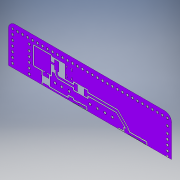
# Autodesk Inventor part: BaseBandAmp_Top_SolderMaskUpper
Saved by Autodesk Inventor 2018 (Build 220112000, 112)
## iProperties
Created: 2018-03-29
Part Number: BaseBandAmp_Top_SolderMaskUpper
Material: Generic
Document SubType Name: Modeling
Designer: Eric Weeks
Density: 1 g/cm^3
Appearance: Default
Author: Eric Weeks
Autodesk Inventor part; units mm, degrees
(part 1 of 2)
ref_plane "YZ Plane" through (0, 0, 0) normal (1, 0, 0) x (0, 1, 0)
ref_plane "XZ Plane" through (0, 0, 0) normal (0, 1, 0) x (-1, 0, 0)
ref_plane "XY Plane" through (0, 0, 0) normal (0, 0, 1) x (1, 0, 0)
sketch "Sketch1" plane through (0, 0, 0) normal (0, 0, 1) x (1, 0, 0)
  line L0 (3476.498, -1500.378) -> (3473.6532, -1500.378) projected
  line L1 (3473.6532, -1500.378) -> (3473.6532, -1503.3396) projected
  line L2 (3473.6532, -1503.3396) -> (3473.9326, -1503.6038) projected
  line L3 (3473.9326, -1503.6038) -> (3477.133, -1503.6038) projected
  line L4 (3477.133, -1503.6038) -> (3478.3268, -1503.1136) projected
  line L5 (3478.3268, -1503.1136) -> (3479.2412, -1502.2043) projected
  line L6 (3479.2412, -1502.2043) -> (3479.7238, -1501.0206) projected
  line L7 (3479.7238, -1501.0206) -> (3479.7238, -1494.0001) projected
  line L8 (3479.7238, -1494.0001) -> (3479.4698, -1493.7359) projected
  line L9 (3479.4698, -1493.7359) -> (3476.498, -1493.7359) projected
  line L10 (3476.498, -1493.7359) -> (3476.498, -1500.378) projected
  line L11 (3455.4922, -1494.0001) -> (3455.4922, -1501.0206) projected
  line L12 (3455.4922, -1501.0206) -> (3455.9748, -1502.2043) projected
  line L13 (3455.9748, -1502.2043) -> (3456.8892, -1503.1136) projected
  line L14 (3456.8892, -1503.1136) -> (3458.083, -1503.6038) projected
  line L15 (3458.083, -1503.6038) -> (3461.2834, -1503.6038) projected
  line L16 (3461.2834, -1503.6038) -> (3461.5374, -1503.3396) projected
  line L17 (3461.5374, -1503.3396) -> (3461.5374, -1500.378) projected
  line L18 (3461.5374, -1500.378) -> (3458.718, -1500.378) projected
  line L19 (3458.718, -1500.378) -> (3458.718, -1493.7359) projected
  line L20 (3458.718, -1493.7359) -> (3455.7462, -1493.7359) projected
  line L21 (3455.7462, -1493.7359) -> (3455.4922, -1494.0001) projected
  line L22 (3770.6966, -1575.7959) -> (3770.9348, -1574.6146) projected
  line L23 (3770.9348, -1574.6146) -> (3770.9348, -1567.3146) projected
  line L24 (3770.9348, -1567.3146) -> (3770.503, -1565.1734) projected
  line L25 (3770.503, -1565.1734) -> (3769.3854, -1563.4919) projected
  line L26 (3769.3854, -1563.4919) -> (3767.709, -1562.3692) projected
  line L27 (3767.709, -1562.3692) -> (3765.5754, -1561.9425) projected
  line L28 (3765.5754, -1561.9425) -> (3756.9902, -1561.9425) projected
  line L29 (3756.9902, -1561.9425) -> (3754.8566, -1562.3692) projected
  line L30 (3754.8566, -1562.3692) -> (3754.755, -1562.4378) projected
  line L31 (3754.755, -1562.4378) -> (3754.5772, -1562.5166) projected
  line L32 (3754.5772, -1562.5166) -> (3754.3994, -1562.6131) projected
  line L33 (3754.3994, -1562.6131) -> (3754.3232, -1562.6283) projected
  line L34 (3754.3232, -1562.6283) -> (3754.247, -1562.6639) projected
  line L35 (3754.247, -1562.6639) -> (3754.0438, -1562.6766) projected
  line L36 (3754.0438, -1562.6766) -> (3753.866, -1562.7096) projected
  line L37 (3753.866, -1562.7096) -> (3749.3448, -1562.7096) projected
  line L38 (3749.3448, -1562.7096) -> (3749.167, -1562.6766) projected
  line L39 (3749.167, -1562.6766) -> (3748.9638, -1562.6639) projected
  line L40 (3748.9638, -1562.6639) -> (3748.8876, -1562.6283) projected
  line L41 (3748.8876, -1562.6283) -> (3748.8114, -1562.6131) projected
  line L42 (3748.8114, -1562.6131) -> (3748.6336, -1562.5166) projected
  line L43 (3748.6336, -1562.5166) -> (3748.4558, -1562.4378) projected
  line L44 (3748.4558, -1562.4378) -> (3748.3542, -1562.3692) projected
  line L45 (3748.3542, -1562.3692) -> (3746.2206, -1561.9425) projected
  line L46 (3746.2206, -1561.9425) -> (3737.6354, -1561.9425) projected
  line L47 (3737.6354, -1561.9425) -> (3735.5018, -1562.3692) projected
  line L48 (3735.5018, -1562.3692) -> (3735.4002, -1562.4378) projected
  line L49 (3735.4002, -1562.4378) -> (3735.2224, -1562.5166) projected
  line L50 (3735.2224, -1562.5166) -> (3735.0446, -1562.6131) projected
  line L51 (3735.0446, -1562.6131) -> (3734.9684, -1562.6283) projected
  line L52 (3734.9684, -1562.6283) -> (3734.8922, -1562.6639) projected
  line L53 (3734.8922, -1562.6639) -> (3734.689, -1562.6766) projected
  line L54 (3734.689, -1562.6766) -> (3734.5112, -1562.7096) projected
  line L55 (3734.5112, -1562.7096) -> (3704.844, -1562.7096) projected
  line L56 (3704.844, -1562.7096) -> (3704.59, -1562.6639) projected
  line L57 (3704.59, -1562.6639) -> (3704.336, -1562.6232) projected
  line L58 (3704.336, -1562.6232) -> (3704.3106, -1562.6156) projected
  line L59 (3704.3106, -1562.6156) -> (3704.2852, -1562.6131) projected
  line L60 (3704.2852, -1562.6131) -> (3704.0566, -1562.481) projected
  line L61 (3704.0566, -1562.481) -> (3703.828, -1562.354) projected
  line L62 (3703.828, -1562.354) -> (3703.828, -1562.3413) projected
  line L63 (3703.828, -1562.3413) -> (3703.8026, -1562.3311) projected
  line L64 (3703.8026, -1562.3311) -> (3703.6502, -1562.1305) projected
  line L65 (3703.6502, -1562.1305) -> (3703.4724, -1561.9324) projected
  line L66 (3703.4724, -1561.9324) -> (3703.447, -1561.9171) projected
  line L67 (3703.447, -1561.9171) -> (3703.447, -1561.9019) projected
  line L68 (3703.447, -1561.9019) -> (3703.3708, -1561.6555) projected
  line L69 (3703.3708, -1561.6555) -> (3703.2692, -1561.4117) projected
  line L70 (3703.2692, -1561.4117) -> (3703.1676, -1560.9189) projected
  line L71 (3703.1676, -1560.9189) -> (3702.05, -1559.2374) projected
  line L72 (3702.05, -1559.2374) -> (3700.3736, -1558.1147) projected
  line L73 (3700.3736, -1558.1147) -> (3700.0434, -1558.0512) projected
  line L74 (3700.0434, -1558.0512) -> (3699.9418, -1558.0131) projected
  line L75 (3699.9418, -1558.0131) -> (3699.8402, -1557.9979) projected
  line L76 (3699.8402, -1557.9979) -> (3699.6878, -1557.9115) projected
  line L77 (3699.6878, -1557.9115) -> (3699.5354, -1557.848) projected
  line L78 (3699.5354, -1557.848) -> (3699.4338, -1557.7795) projected
  line L79 (3699.4338, -1557.7795) -> (3699.3576, -1557.7287) projected
  line L80 (3699.3576, -1557.7287) -> (3699.2306, -1557.5966) projected
  line L81 (3699.2306, -1557.5966) -> (3699.1036, -1557.4797) projected
  line L82 (3699.1036, -1557.4797) -> (3699.0528, -1557.3858) projected
  line L83 (3699.0528, -1557.3858) -> (3698.9766, -1557.307) projected
  line L84 (3698.9766, -1557.307) -> (3698.9258, -1557.1419) projected
  line L85 (3698.9258, -1557.1419) -> (3698.8242, -1556.9895) projected
  line L86 (3698.8242, -1556.9895) -> (3698.8242, -1556.8828) projected
  line L87 (3698.8242, -1556.8828) -> (3698.7734, -1556.7838) projected
  line L88 (3698.7734, -1556.7838) -> (3698.0876, -1553.3294) projected
  line L89 (3698.0876, -1553.3294) -> (3696.6398, -1551.1551) projected
  line L90 (3696.6398, -1551.1551) -> (3696.2588, -1550.5989) projected
  line L91 (3696.2588, -1550.5989) -> (3695.7, -1550.2255) projected
  line L92 (3695.7, -1550.2255) -> (3695.5984, -1550.1163) projected
  line L93 (3695.5984, -1550.1163) -> (3695.4714, -1550.0248) projected
  line L94 (3695.4714, -1550.0248) -> (3659.632, -1514.2007) projected
  line L95 (3659.632, -1514.2007) -> (3659.5558, -1514.0711) projected
  line L96 (3659.5558, -1514.0711) -> (3659.4288, -1513.9568) projected
  line L97 (3659.4288, -1513.9568) -> (3659.0732, -1513.4006) projected
  line L98 (3659.0732, -1513.4006) -> (3656.33, -1511.5769) projected
  line L99 (3656.33, -1511.5769) -> (3653.7646, -1511.0663) projected
  line L100 (3653.7646, -1511.0663) -> (3653.1042, -1510.9342) projected
  line L101 (3653.1042, -1510.9342) -> (3652.4692, -1511.0663) projected
  line L102 (3652.4692, -1511.0663) -> (3652.2914, -1511.0689) projected
  line L103 (3652.2914, -1511.0689) -> (3652.139, -1511.0968) projected
  line L104 (3652.139, -1511.0968) -> (3544.824, -1511.0968) projected
  line L105 (3544.824, -1511.0968) -> (3544.6716, -1511.0714) projected
  line L106 (3544.6716, -1511.0714) -> (3544.5446, -1511.0714) projected
  line L107 (3544.5446, -1511.0714) -> (3544.3922, -1511.0231) projected
  line L108 (3544.3922, -1511.0231) -> (3544.2652, -1511.0003) projected
  line L109 (3544.2652, -1511.0003) -> (3544.1382, -1510.9292) projected
  line L110 (3544.1382, -1510.9292) -> (3544.0112, -1510.8809) projected
  line L111 (3544.0112, -1510.8809) -> (3543.9096, -1510.7895) projected
  line L112 (3543.9096, -1510.7895) -> (3543.7826, -1510.7183) projected
  line L113 (3543.7826, -1510.7183) -> (3543.681, -1510.6117) projected
  line L114 (3543.681, -1510.6117) -> (3543.5794, -1510.5202) projected
  line L115 (3543.5794, -1510.5202) -> (3543.5032, -1510.3983) projected
  line L116 (3543.5032, -1510.3983) -> (3543.427, -1510.2891) projected
  line L117 (3543.427, -1510.2891) -> (3543.3762, -1510.157) projected
  line L118 (3543.3762, -1510.157) -> (3543.3, -1510.0351) projected
  line L119 (3543.3, -1510.0351) -> (3543.2746, -1509.8954) projected
  line L120 (3543.2746, -1509.8954) -> (3543.2238, -1509.7633) projected
  line L121 (3543.2238, -1509.7633) -> (3543.2238, -1509.6236) projected
  line L122 (3543.2238, -1509.6236) -> (3543.1984, -1509.4839) projected
  line L123 (3543.1984, -1509.4839) -> (3543.1984, -1508.0818) projected
  line L124 (3543.1984, -1508.0818) -> (3542.7666, -1505.9406) projected
  line L125 (3542.7666, -1505.9406) -> (3541.649, -1504.2591) projected
  line L126 (3541.649, -1504.2591) -> (3539.9726, -1503.1364) projected
  line L127 (3539.9726, -1503.1364) -> (3537.839, -1502.7097) projected
  line L128 (3537.839, -1502.7097) -> (3525.4438, -1502.7097) projected
  line L129 (3525.4438, -1502.7097) -> (3523.0308, -1503.1923) projected
  line L130 (3523.0308, -1503.1923) -> (3522.8784, -1503.1949) projected
  line L131 (3522.8784, -1503.1949) -> (3522.726, -1503.2228) projected
  line L132 (3522.726, -1503.2228) -> (3502.4568, -1503.2228) projected
  line L133 (3502.4568, -1503.2228) -> (3502.3044, -1503.1949) projected
  line L134 (3502.3044, -1503.1949) -> (3502.152, -1503.1923) projected
  line L135 (3502.152, -1503.1923) -> (3499.739, -1502.7097) projected
  line L136 (3499.739, -1502.7097) -> (3487.3438, -1502.7097) projected
  line L137 (3487.3438, -1502.7097) -> (3485.2102, -1503.1364) projected
  line L138 (3485.2102, -1503.1364) -> (3483.5338, -1504.2591) projected
  line L139 (3483.5338, -1504.2591) -> (3482.4162, -1505.9406) projected
  line L140 (3482.4162, -1505.9406) -> (3481.9844, -1508.0818) projected
  line L141 (3481.9844, -1508.0818) -> (3481.9844, -1509.4839) projected
  line L142 (3481.9844, -1509.4839) -> (3481.959, -1509.6236) projected
  line L143 (3481.959, -1509.6236) -> (3481.959, -1509.7633) projected
  line L144 (3481.959, -1509.7633) -> (3481.9082, -1509.8954) projected
  line L145 (3481.9082, -1509.8954) -> (3481.8828, -1510.0351) projected
  line L146 (3481.8828, -1510.0351) -> (3481.8066, -1510.157) projected
  line L147 (3481.8066, -1510.157) -> (3481.7558, -1510.2891) projected
  line L148 (3481.7558, -1510.2891) -> (3481.6796, -1510.3983) projected
  line L149 (3481.6796, -1510.3983) -> (3481.6034, -1510.5202) projected
  line L150 (3481.6034, -1510.5202) -> (3481.5018, -1510.6117) projected
  line L151 (3481.5018, -1510.6117) -> (3481.4002, -1510.7183) projected
  line L152 (3481.4002, -1510.7183) -> (3481.2732, -1510.7895) projected
  line L153 (3481.2732, -1510.7895) -> (3481.1716, -1510.8809) projected
  line L154 (3481.1716, -1510.8809) -> (3481.0446, -1510.9292) projected
  line L155 (3481.0446, -1510.9292) -> (3480.9176, -1511.0003) projected
  line L156 (3480.9176, -1511.0003) -> (3480.7906, -1511.0231) projected
  line L157 (3480.7906, -1511.0231) -> (3480.6382, -1511.0714) projected
  line L158 (3480.6382, -1511.0714) -> (3480.5112, -1511.0714) projected
  line L159 (3480.5112, -1511.0714) -> (3480.3588, -1511.0968) projected
  line L160 (3480.3588, -1511.0968) -> (3453.2062, -1511.0968) projected
  line L161 (3453.2062, -1511.0968) -> (3453.0792, -1511.0714) projected
  line L162 (3453.0792, -1511.0714) -> (3452.9268, -1511.0714) projected
  line L163 (3452.9268, -1511.0714) -> (3452.7998, -1511.0231) projected
  line L164 (3452.7998, -1511.0231) -> (3452.6728, -1511.0003) projected
  line L165 (3452.6728, -1511.0003) -> (3452.5458, -1510.9292) projected
  line L166 (3452.5458, -1510.9292) -> (3452.4188, -1510.8809) projected
  line L167 (3452.4188, -1510.8809) -> (3452.2918, -1510.7895) projected
  line L168 (3452.2918, -1510.7895) -> (3452.1902, -1510.7183) projected
  line L169 (3452.1902, -1510.7183) -> (3452.0886, -1510.6117) projected
  line L170 (3452.0886, -1510.6117) -> (3451.987, -1510.5202) projected
  line L171 (3451.987, -1510.5202) -> (3451.9108, -1510.3983) projected
  line L172 (3451.9108, -1510.3983) -> (3451.8346, -1510.2891) projected
  line L173 (3451.8346, -1510.2891) -> (3451.7838, -1510.157) projected
  line L174 (3451.7838, -1510.157) -> (3451.7076, -1510.0351) projected
  line L175 (3451.7076, -1510.0351) -> (3451.6822, -1509.8954) projected
  line L176 (3451.6822, -1509.8954) -> (3451.6314, -1509.7633) projected
  line L177 (3451.6314, -1509.7633) -> (3451.6314, -1509.6236) projected
  line L178 (3451.6314, -1509.6236) -> (3451.606, -1509.4839) projected
  line L179 (3451.606, -1509.4839) -> (3451.606, -1461.4474) projected
  line L180 (3451.606, -1461.4474) -> (3451.5806, -1461.3128) projected
  line L181 (3451.5806, -1461.3128) -> (3451.4536, -1461.2874) projected
  line L182 (3451.4536, -1461.2874) -> (3403.2698, -1461.2874) projected
  line L183 (3403.2698, -1461.2874) -> (3403.0158, -1461.2417) projected
  line L184 (3403.0158, -1461.2417) -> (3402.7618, -1461.201) projected
  line L185 (3402.7618, -1461.201) -> (3402.7364, -1461.1934) projected
  line L186 (3402.7364, -1461.1934) -> (3402.711, -1461.1909) projected
  line L187 (3402.711, -1461.1909) -> (3402.4824, -1461.0588) projected
  line L188 (3402.4824, -1461.0588) -> (3402.2538, -1460.9318) projected
  line L189 (3402.2538, -1460.9318) -> (3402.2538, -1460.9191) projected
  line L190 (3402.2538, -1460.9191) -> (3402.2284, -1460.9089) projected
  line L191 (3402.2284, -1460.9089) -> (3402.076, -1460.7083) projected
  line L192 (3402.076, -1460.7083) -> (3401.8982, -1460.5102) projected
  line L193 (3401.8982, -1460.5102) -> (3401.8728, -1460.4949) projected
  line L194 (3401.8728, -1460.4949) -> (3401.8728, -1460.4797) projected
  line L195 (3401.8728, -1460.4797) -> (3401.7712, -1460.2333) projected
  line L196 (3401.7712, -1460.2333) -> (3401.695, -1459.9895) projected
  line L197 (3401.695, -1459.9895) -> (3401.5426, -1459.3062) projected
  line L198 (3401.5426, -1459.3062) -> (3400.425, -1457.6247) projected
  line L199 (3400.425, -1457.6247) -> (3398.7486, -1456.502) projected
  line L200 (3398.7486, -1456.502) -> (3396.615, -1456.0753) projected
  line L201 (3396.615, -1456.0753) -> (3332.4038, -1456.0753) projected
  line L202 (3332.4038, -1456.0753) -> (3330.2702, -1456.502) projected
  line L203 (3330.2702, -1456.502) -> (3328.5938, -1457.6247) projected
  line L204 (3328.5938, -1457.6247) -> (3327.4762, -1459.3062) projected
  line L205 (3327.4762, -1459.3062) -> (3327.0444, -1461.4474) projected
  line L206 (3327.0444, -1461.4474) -> (3327.0444, -1525.6434) projected
  line L207 (3327.0444, -1525.6434) -> (3327.4762, -1527.7846) projected
  line L208 (3327.4762, -1527.7846) -> (3328.5938, -1529.4661) projected
  line L209 (3328.5938, -1529.4661) -> (3330.2702, -1530.5888) projected
  line L210 (3330.2702, -1530.5888) -> (3332.4038, -1531.0155) projected
  line L211 (3332.4038, -1531.0155) -> (3359.15, -1531.0155) projected
  line L212 (3359.15, -1531.0155) -> (3359.3024, -1531.0383) projected
  line L213 (3359.3024, -1531.0383) -> (3359.4294, -1531.0383) projected
  line L214 (3359.4294, -1531.0383) -> (3359.5818, -1531.0866) projected
  line L215 (3359.5818, -1531.0866) -> (3359.7088, -1531.112) projected
  line L216 (3359.7088, -1531.112) -> (3359.8358, -1531.1831) projected
  line L217 (3359.8358, -1531.1831) -> (3359.9628, -1531.2314) projected
  line L218 (3359.9628, -1531.2314) -> (3360.0644, -1531.3203) projected
  line L219 (3360.0644, -1531.3203) -> (3360.1914, -1531.3914) projected
  line L220 (3360.1914, -1531.3914) -> (3360.293, -1531.5006) projected
  line L221 (3360.293, -1531.5006) -> (3360.3946, -1531.5895) projected
  line L222 (3360.3946, -1531.5895) -> (3360.4708, -1531.714) projected
  line L223 (3360.4708, -1531.714) -> (3360.547, -1531.8207) projected
  line L224 (3360.547, -1531.8207) -> (3360.5978, -1531.9527) projected
  line L225 (3360.5978, -1531.9527) -> (3360.674, -1532.0747) projected
  line L226 (3360.674, -1532.0747) -> (3360.6994, -1532.2144) projected
  line L227 (3360.6994, -1532.2144) -> (3360.7502, -1532.3464) projected
  line L228 (3360.7502, -1532.3464) -> (3360.7502, -1532.4887) projected
  line L229 (3360.7502, -1532.4887) -> (3360.7756, -1532.6284) projected
  line L230 (3360.7756, -1532.6284) -> (3360.7756, -1541.9756) projected
  line L231 (3360.7756, -1541.9756) -> (3361.2582, -1544.3962) projected
  line L232 (3361.2582, -1544.3962) -> (3361.2582, -1544.5537) projected
  line L233 (3361.2582, -1544.5537) -> (3361.2836, -1544.7112) projected
  line L234 (3361.2836, -1544.7112) -> (3361.2836, -1564.96) projected
  line L235 (3361.2836, -1564.96) -> (3361.2582, -1565.1175) projected
  line L236 (3361.2582, -1565.1175) -> (3361.2582, -1565.275) projected
  line L237 (3361.2582, -1565.275) -> (3360.7756, -1567.6956) projected
  line L238 (3360.7756, -1567.6956) -> (3360.7756, -1575.7959) projected
  line L239 (3410.458, -1480.693) -> (3410.458, -1467.358) projected
  line L240 (3410.458, -1467.358) -> (3428.238, -1467.358) projected
  line L241 (3428.238, -1467.358) -> (3428.238, -1500.378) projected
  line L242 (3428.238, -1500.378) -> (3422.523, -1500.378) projected
  line L243 (3422.523, -1500.378) -> (3422.523, -1511.5845) projected
  line L244 (3422.523, -1511.5845) -> (3427.1204, -1516.1768) projected
  line L245 (3427.1204, -1516.1768) -> (3487.1914, -1516.1768) projected
  line L246 (3487.1914, -1516.1768) -> (3487.1914, -1507.9218) projected
  line L247 (3487.1914, -1507.9218) -> (3499.8914, -1507.9218) projected
  line L248 (3499.8914, -1507.9218) -> (3499.8914, -1530.7818) projected
  line L249 (3499.8914, -1530.7818) -> (3487.1914, -1530.7818) projected
  line L250 (3487.1914, -1530.7818) -> (3487.1914, -1522.5268) projected
  line L251 (3487.1914, -1522.5268) -> (3425.7234, -1522.5268) projected
  line L252 (3425.7234, -1522.5268) -> (3425.6726, -1522.5141) projected
  line L253 (3425.6726, -1522.5141) -> (3425.5202, -1522.5268) projected
  line L254 (3425.5202, -1522.5268) -> (3425.1138, -1522.4201) projected
  line L255 (3425.1138, -1522.4201) -> (3424.7074, -1522.3465) projected
  line L256 (3424.7074, -1522.3465) -> (3424.5804, -1522.2753) projected
  line L257 (3424.5804, -1522.2753) -> (3424.4534, -1522.2398) projected
  line L258 (3424.4534, -1522.2398) -> (3424.1232, -1522.001) projected
  line L259 (3424.1232, -1522.001) -> (3423.7422, -1521.7927) projected
  line L260 (3423.7422, -1521.7927) -> (3423.666, -1521.6861) projected
  line L261 (3423.666, -1521.6861) -> (3423.6152, -1521.6454) projected
  line L262 (3423.6152, -1521.6454) -> (3417.062, -1515.0973) projected
  line L263 (3417.062, -1515.0973) -> (3417.0112, -1515.0389) projected
  line L264 (3417.0112, -1515.0389) -> (3416.9096, -1514.95) projected
  line L265 (3416.9096, -1514.95) -> (3416.7064, -1514.5893) projected
  line L266 (3416.7064, -1514.5893) -> (3416.4524, -1514.2464) projected
  line L267 (3416.4524, -1514.2464) -> (3416.427, -1514.1118) projected
  line L268 (3416.427, -1514.1118) -> (3416.3508, -1513.9899) projected
  line L269 (3416.3508, -1513.9899) -> (3416.2746, -1513.5809) projected
  line L270 (3416.2746, -1513.5809) -> (3416.173, -1513.1771) projected
  line L271 (3416.173, -1513.1771) -> (3416.173, -1513.0374) projected
  line L272 (3416.173, -1513.0374) -> (3416.173, -1512.9688) projected
  line L273 (3416.173, -1512.9688) -> (3416.173, -1500.378) projected
  line L274 (3416.173, -1500.378) -> (3410.458, -1500.378) projected
  line L275 (3410.458, -1500.378) -> (3410.458, -1487.043) projected
  line L276 (3410.458, -1487.043) -> (3396.7674, -1487.043) projected
  line L277 (3396.7674, -1487.043) -> (3396.7674, -1525.8034) projected
  line L278 (3396.7674, -1525.8034) -> (3380.5876, -1525.8034) projected
  line L279 (3380.5876, -1525.8034) -> (3380.5876, -1529.4356) projected
  line L280 (3380.5876, -1529.4356) -> (3388.8426, -1529.4356) projected
  line L281 (3388.8426, -1529.4356) -> (3388.8426, -1542.1356) projected
  line L282 (3388.8426, -1542.1356) -> (3365.9826, -1542.1356) projected
  line L283 (3365.9826, -1542.1356) -> (3365.9826, -1529.4356) projected
  line L284 (3365.9826, -1529.4356) -> (3374.2376, -1529.4356) projected
  line L285 (3374.2376, -1529.4356) -> (3374.2376, -1525.8034) projected
  line L286 (3374.2376, -1525.8034) -> (3332.2514, -1525.8034) projected
  line L287 (3332.2514, -1525.8034) -> (3332.2514, -1461.2874) projected
  line L288 (3332.2514, -1461.2874) -> (3396.7674, -1461.2874) projected
  line L289 (3396.7674, -1461.2874) -> (3396.7674, -1480.693) projected
  line L290 (3396.7674, -1480.693) -> (3410.458, -1480.693) projected
  line L291 (3658.0831, -1575.7959) -> (3658.0572, -1571.1246) projected
  line L292 (3658.0572, -1571.1246) -> (3658.0826, -1570.9925) projected
  line L293 (3658.0826, -1570.9925) -> (3658.2096, -1570.9646) projected
  line L294 (3658.2096, -1570.9646) -> (3675.4308, -1570.9646) projected
  line L295 (3675.4308, -1570.9646) -> (3675.5578, -1570.9392) projected
  line L296 (3675.5578, -1570.9392) -> (3675.7102, -1570.9392) projected
  line L297 (3675.7102, -1570.9392) -> (3675.8372, -1570.8909) projected
  line L298 (3675.8372, -1570.8909) -> (3675.9896, -1570.8681) projected
  line L299 (3675.9896, -1570.8681) -> (3676.0912, -1570.797) projected
  line L300 (3676.0912, -1570.797) -> (3676.2436, -1570.7487) projected
  line L301 (3676.2436, -1570.7487) -> (3676.3452, -1570.6573) projected
  line L302 (3676.3452, -1570.6573) -> (3676.4722, -1570.5861) projected
  line L303 (3676.4722, -1570.5861) -> (3676.5484, -1570.4795) projected
  line L304 (3676.5484, -1570.4795) -> (3676.65, -1570.388) projected
  line L305 (3676.65, -1570.388) -> (3676.7262, -1570.2661) projected
  line L306 (3676.7262, -1570.2661) -> (3676.8278, -1570.1569) projected
  line L307 (3676.8278, -1570.1569) -> (3676.8786, -1570.0248) projected
  line L308 (3676.8786, -1570.0248) -> (3676.9548, -1569.9029) projected
  line L309 (3676.9548, -1569.9029) -> (3676.9548, -1569.7632) projected
  line L310 (3676.9548, -1569.7632) -> (3677.0056, -1569.6311) projected
  line L311 (3677.0056, -1569.6311) -> (3677.0056, -1569.4914) projected
  line L312 (3677.0056, -1569.4914) -> (3677.031, -1569.3517) projected
  line L313 (3677.031, -1569.3517) -> (3677.031, -1563.0601) projected
  line L314 (3677.031, -1563.0601) -> (3677.4628, -1560.9189) projected
  line L315 (3677.4628, -1560.9189) -> (3678.5804, -1559.2374) projected
  line L316 (3678.5804, -1559.2374) -> (3678.6058, -1559.2323) projected
  line L317 (3678.6058, -1559.2323) -> (3678.6058, -1559.2196) projected
  line L318 (3678.6058, -1559.2196) -> (3678.6312, -1559.212) projected
  line L319 (3678.6312, -1559.212) -> (3678.809, -1559.0266) projected
  line L320 (3678.809, -1559.0266) -> (3679.0122, -1558.8437) projected
  line L321 (3679.0122, -1558.8437) -> (3679.0122, -1558.8285) projected
  line L322 (3679.0122, -1558.8285) -> (3679.0122, -1558.8158) projected
  line L323 (3679.0122, -1558.8158) -> (3679.1392, -1558.577) projected
  line L324 (3679.1392, -1558.577) -> (3679.2408, -1558.3433) projected
  line L325 (3679.2408, -1558.3433) -> (3679.2408, -1558.3256) projected
  line L326 (3679.2408, -1558.3256) -> (3679.2662, -1558.3078) projected
  line L327 (3679.2662, -1558.3078) -> (3679.2916, -1558.0462) projected
  line L328 (3679.2916, -1558.0462) -> (3679.317, -1557.7845) projected
  line L329 (3679.317, -1557.7845) -> (3679.317, -1557.7668) projected
  line L330 (3679.317, -1557.7668) -> (3679.317, -1557.7515) projected
  line L331 (3679.317, -1557.7515) -> (3679.2408, -1557.4975) projected
  line L332 (3679.2408, -1557.4975) -> (3679.1646, -1557.241) projected
  line L333 (3679.1646, -1557.241) -> (3679.1646, -1557.2257) projected
  line L334 (3679.1646, -1557.2257) -> (3679.1646, -1557.208) projected
  line L335 (3679.1646, -1557.208) -> (3679.0122, -1556.9946) projected
  line L336 (3679.0122, -1556.9946) -> (3678.8598, -1556.7762) projected
  line L337 (3678.8598, -1556.7762) -> (3678.8598, -1556.766) projected
  line L338 (3678.8598, -1556.766) -> (3678.8344, -1556.7508) projected
  line L339 (3678.8344, -1556.7508) -> (3650.1578, -1528.0792) projected
  line L340 (3650.1578, -1528.0792) -> (3650.107, -1528.0386) projected
  line L341 (3650.107, -1528.0386) -> (3650.0562, -1527.9853) projected
  line L342 (3650.0562, -1527.9853) -> (3649.8784, -1527.8786) projected
  line L343 (3649.8784, -1527.8786) -> (3649.7006, -1527.7567) projected
  line L344 (3649.7006, -1527.7567) -> (3649.6498, -1527.7389) projected
  line L345 (3649.6498, -1527.7389) -> (3649.5736, -1527.7033) projected
  line L346 (3649.5736, -1527.7033) -> (3649.3704, -1527.6678) projected
  line L347 (3649.3704, -1527.6678) -> (3649.1672, -1527.6119) projected
  line L348 (3649.1672, -1527.6119) -> (3649.091, -1527.6195) projected
  line L349 (3649.091, -1527.6195) -> (3649.0402, -1527.6068) projected
  line L350 (3649.0402, -1527.6068) -> (3544.824, -1527.6068) projected
  line L351 (3544.824, -1527.6068) -> (3544.6716, -1527.6322) projected
  line L352 (3544.6716, -1527.6322) -> (3544.5446, -1527.6322) projected
  line L353 (3544.5446, -1527.6322) -> (3544.3922, -1527.6805) projected
  line L354 (3544.3922, -1527.6805) -> (3544.2652, -1527.7033) projected
  line L355 (3544.2652, -1527.7033) -> (3544.1382, -1527.7744) projected
  line L356 (3544.1382, -1527.7744) -> (3544.0112, -1527.8227) projected
  line L357 (3544.0112, -1527.8227) -> (3543.9096, -1527.9141) projected
  line L358 (3543.9096, -1527.9141) -> (3543.7826, -1527.9853) projected
  line L359 (3543.7826, -1527.9853) -> (3543.681, -1528.0919) projected
  line L360 (3543.681, -1528.0919) -> (3543.5794, -1528.1834) projected
  line L361 (3543.5794, -1528.1834) -> (3543.5032, -1528.3053) projected
  line L362 (3543.5032, -1528.3053) -> (3543.427, -1528.412) projected
  line L363 (3543.427, -1528.412) -> (3543.3762, -1528.5466) projected
  line L364 (3543.3762, -1528.5466) -> (3543.3, -1528.6685) projected
  line L365 (3543.3, -1528.6685) -> (3543.2746, -1528.8082) projected
  line L366 (3543.2746, -1528.8082) -> (3543.2238, -1528.9403) projected
  line L367 (3543.2238, -1528.9403) -> (3543.2238, -1529.08) projected
  line L368 (3543.2238, -1529.08) -> (3543.1984, -1529.2197) projected
  line L369 (3543.1984, -1529.2197) -> (3543.1984, -1530.6218) projected
  line L370 (3543.1984, -1530.6218) -> (3542.7666, -1532.763) projected
  line L371 (3542.7666, -1532.763) -> (3541.649, -1534.4445) projected
  line L372 (3541.649, -1534.4445) -> (3539.9726, -1535.5672) projected
  line L373 (3539.9726, -1535.5672) -> (3537.839, -1535.9939) projected
  line L374 (3537.839, -1535.9939) -> (3525.4438, -1535.9939) projected
  line L375 (3525.4438, -1535.9939) -> (3523.0308, -1535.5113) projected
  line L376 (3523.0308, -1535.5113) -> (3522.8784, -1535.5087) projected
  line L377 (3522.8784, -1535.5087) -> (3522.726, -1535.4808) projected
  line L378 (3522.726, -1535.4808) -> (3502.4568, -1535.4808) projected
  line L379 (3502.4568, -1535.4808) -> (3502.3044, -1535.5087) projected
  line L380 (3502.3044, -1535.5087) -> (3502.152, -1535.5113) projected
  line L381 (3502.152, -1535.5113) -> (3499.739, -1535.9939) projected
  line L382 (3499.739, -1535.9939) -> (3487.3438, -1535.9939) projected
  line L383 (3487.3438, -1535.9939) -> (3485.2102, -1535.5672) projected
  line L384 (3485.2102, -1535.5672) -> (3483.5338, -1534.4445) projected
  line L385 (3483.5338, -1534.4445) -> (3482.4162, -1532.763) projected
  line L386 (3482.4162, -1532.763) -> (3481.9844, -1530.6218) projected
  line L387 (3481.9844, -1530.6218) -> (3481.9844, -1529.2197) projected
  line L388 (3481.9844, -1529.2197) -> (3481.959, -1529.08) projected
  line L389 (3481.959, -1529.08) -> (3481.959, -1528.9403) projected
  line L390 (3481.959, -1528.9403) -> (3481.9082, -1528.8082) projected
  line L391 (3481.9082, -1528.8082) -> (3481.8828, -1528.6685) projected
  line L392 (3481.8828, -1528.6685) -> (3481.8066, -1528.5466) projected
  line L393 (3481.8066, -1528.5466) -> (3481.7558, -1528.412) projected
  line L394 (3481.7558, -1528.412) -> (3481.6796, -1528.3053) projected
  line L395 (3481.6796, -1528.3053) -> (3481.6034, -1528.1834) projected
  line L396 (3481.6034, -1528.1834) -> (3481.5018, -1528.0919) projected
  line L397 (3481.5018, -1528.0919) -> (3481.4002, -1527.9853) projected
  line L398 (3481.4002, -1527.9853) -> (3481.2732, -1527.9141) projected
  line L399 (3481.2732, -1527.9141) -> (3481.1716, -1527.8227) projected
  line L400 (3481.1716, -1527.8227) -> (3481.0446, -1527.7744) projected
  line L401 (3481.0446, -1527.7744) -> (3480.9176, -1527.7033) projected
  line L402 (3480.9176, -1527.7033) -> (3480.7906, -1527.6805) projected
  line L403 (3480.7906, -1527.6805) -> (3480.6382, -1527.6322) projected
  line L404 (3480.6382, -1527.6322) -> (3480.5112, -1527.6322) projected
  line L405 (3480.5112, -1527.6322) -> (3480.3588, -1527.6068) projected
  line L406 (3480.3588, -1527.6068) -> (3426.7648, -1527.6068) projected
  line L407 (3426.7648, -1527.6068) -> (3426.6124, -1527.6347) projected
  line L408 (3426.6124, -1527.6347) -> (3426.46, -1527.6373) projected
  line L409 (3426.46, -1527.6373) -> (3425.7996, -1527.7694) projected
  line L410 (3425.7996, -1527.7694) -> (3425.1392, -1527.6373) projected
  line L411 (3425.1392, -1527.6373) -> (3422.5738, -1527.1267) projected
  line L412 (3422.5738, -1527.1267) -> (3419.856, -1525.303) projected
  line L413 (3419.856, -1525.303) -> (3419.475, -1524.7468) projected
  line L414 (3419.475, -1524.7468) -> (3419.3734, -1524.6325) projected
  line L415 (3419.3734, -1524.6325) -> (3419.2718, -1524.5029) projected
  line L416 (3419.2718, -1524.5029) -> (3414.1918, -1519.4255) projected
  line L417 (3414.1918, -1519.4255) -> (3414.0648, -1519.334) projected
  line L418 (3414.0648, -1519.334) -> (3413.9632, -1519.2248) projected
  line L419 (3413.9632, -1519.2248) -> (3413.4044, -1518.8514) projected
  line L420 (3413.4044, -1518.8514) -> (3411.5756, -1516.1209) projected
  line L421 (3411.5756, -1516.1209) -> (3411.1946, -1514.1981) projected
  line L422 (3411.1946, -1514.1981) -> (3411.093, -1513.9543) projected
  line L423 (3411.093, -1513.9543) -> (3411.0168, -1513.7054) projected
  line L424 (3411.0168, -1513.7054) -> (3410.9914, -1513.6927) projected
  line L425 (3410.9914, -1513.6927) -> (3410.9914, -1513.6774) projected
  line L426 (3410.9914, -1513.6774) -> (3410.8136, -1513.4793) projected
  line L427 (3410.8136, -1513.4793) -> (3410.6358, -1513.2787) projected
  line L428 (3410.6358, -1513.2787) -> (3410.6358, -1513.2685) projected
  line L429 (3410.6358, -1513.2685) -> (3410.6104, -1513.2558) projected
  line L430 (3410.6104, -1513.2558) -> (3410.3818, -1513.1288) projected
  line L431 (3410.3818, -1513.1288) -> (3410.1532, -1512.9942) projected
  line L432 (3410.1532, -1512.9942) -> (3410.1532, -1512.9942) projected
  line L433 (3410.1532, -1512.9942) -> (3410.1278, -1512.9866) projected
  line L434 (3410.1278, -1512.9866) -> (3409.8738, -1512.9459) projected
  line L435 (3409.8738, -1512.9459) -> (3409.6198, -1512.9002) projected
  line L436 (3409.6198, -1512.9002) -> (3403.6, -1512.9002) projected
  line L437 (3403.6, -1512.9002) -> (3403.4476, -1512.9256) projected
  line L438 (3403.4476, -1512.9256) -> (3403.3206, -1512.9256) projected
  line L439 (3403.3206, -1512.9256) -> (3403.1682, -1512.9739) projected
  line L440 (3403.1682, -1512.9739) -> (3403.0412, -1512.9967) projected
  line L441 (3403.0412, -1512.9967) -> (3402.9142, -1513.0678) projected
  line L442 (3402.9142, -1513.0678) -> (3402.7872, -1513.1161) projected
  line L443 (3402.7872, -1513.1161) -> (3402.6856, -1513.2075) projected
  line L444 (3402.6856, -1513.2075) -> (3402.5586, -1513.2787) projected
  line L445 (3402.5586, -1513.2787) -> (3402.457, -1513.3853) projected
  line L446 (3402.457, -1513.3853) -> (3402.3554, -1513.4768) projected
  line L447 (3402.3554, -1513.4768) -> (3402.2792, -1513.5987) projected
  line L448 (3402.2792, -1513.5987) -> (3402.203, -1513.7054) projected
  line L449 (3402.203, -1513.7054) -> (3402.1522, -1513.84) projected
  line L450 (3402.1522, -1513.84) -> (3402.076, -1513.9619) projected
  line L451 (3402.076, -1513.9619) -> (3402.0506, -1514.1016) projected
  line L452 (3402.0506, -1514.1016) -> (3401.9998, -1514.2337) projected
  line L453 (3401.9998, -1514.2337) -> (3401.9998, -1514.3734) projected
  line L454 (3401.9998, -1514.3734) -> (3401.9744, -1514.5131) projected
  line L455 (3401.9744, -1514.5131) -> (3401.9744, -1525.6434) projected
  line L456 (3401.9744, -1525.6434) -> (3401.5426, -1527.7846) projected
  line L457 (3401.5426, -1527.7846) -> (3400.425, -1529.4661) projected
  line L458 (3400.425, -1529.4661) -> (3398.7486, -1530.5888) projected
  line L459 (3398.7486, -1530.5888) -> (3396.615, -1531.0155) projected
  line L460 (3396.615, -1531.0155) -> (3395.6752, -1531.0155) projected
  line L461 (3395.6752, -1531.0155) -> (3395.5228, -1531.0383) projected
  line L462 (3395.5228, -1531.0383) -> (3395.3958, -1531.0383) projected
  line L463 (3395.3958, -1531.0383) -> (3395.2434, -1531.0866) projected
  line L464 (3395.2434, -1531.0866) -> (3395.1164, -1531.112) projected
  line L465 (3395.1164, -1531.112) -> (3394.9894, -1531.1831) projected
  line L466 (3394.9894, -1531.1831) -> (3394.8624, -1531.2314) projected
  line L467 (3394.8624, -1531.2314) -> (3394.7608, -1531.3203) projected
  line L468 (3394.7608, -1531.3203) -> (3394.6338, -1531.3914) projected
  line L469 (3394.6338, -1531.3914) -> (3394.5322, -1531.5006) projected
  line L470 (3394.5322, -1531.5006) -> (3394.4306, -1531.5895) projected
  line L471 (3394.4306, -1531.5895) -> (3394.3544, -1531.714) projected
  line L472 (3394.3544, -1531.714) -> (3394.2782, -1531.8207) projected
  line L473 (3394.2782, -1531.8207) -> (3394.2274, -1531.9527) projected
  line L474 (3394.2274, -1531.9527) -> (3394.1512, -1532.0747) projected
  line L475 (3394.1512, -1532.0747) -> (3394.1258, -1532.2144) projected
  line L476 (3394.1258, -1532.2144) -> (3394.075, -1532.3464) projected
  line L477 (3394.075, -1532.3464) -> (3394.075, -1532.4887) projected
  line L478 (3394.075, -1532.4887) -> (3394.0496, -1532.6284) projected
  line L479 (3394.0496, -1532.6284) -> (3394.0496, -1541.9756) projected
  line L480 (3394.0496, -1541.9756) -> (3393.567, -1544.3962) projected
  line L481 (3393.567, -1544.3962) -> (3393.567, -1544.5537) projected
  line L482 (3393.567, -1544.5537) -> (3393.5416, -1544.7112) projected
  line L483 (3393.5416, -1544.7112) -> (3393.5416, -1564.0177) projected
  line L484 (3393.5416, -1564.0177) -> (3393.567, -1564.1574) projected
  line L485 (3393.567, -1564.1574) -> (3393.567, -1564.2971) projected
  line L486 (3393.567, -1564.2971) -> (3393.6178, -1564.4292) projected
  line L487 (3393.6178, -1564.4292) -> (3393.6432, -1564.5689) projected
  line L488 (3393.6432, -1564.5689) -> (3393.7194, -1564.6908) projected
  line L489 (3393.7194, -1564.6908) -> (3393.7702, -1564.8254) projected
  line L490 (3393.7702, -1564.8254) -> (3393.8464, -1564.9321) projected
  line L491 (3393.8464, -1564.9321) -> (3393.9226, -1565.054) projected
  line L492 (3393.9226, -1565.054) -> (3394.0242, -1565.1455) projected
  line L493 (3394.0242, -1565.1455) -> (3394.1258, -1565.2521) projected
  line L494 (3394.1258, -1565.2521) -> (3394.2274, -1565.3233) projected
  line L495 (3394.2274, -1565.3233) -> (3394.3544, -1565.4147) projected
  line L496 (3394.3544, -1565.4147) -> (3394.4814, -1565.463) projected
  line L497 (3394.4814, -1565.463) -> (3394.6084, -1565.5341) projected
  line L498 (3394.6084, -1565.5341) -> (3394.7354, -1565.5569) projected
  line L499 (3394.7354, -1565.5569) -> (3394.8624, -1565.6052) projected
  line L500 (3394.8624, -1565.6052) -> (3395.0148, -1565.6052) projected
  line L501 (3395.0148, -1565.6052) -> (3395.1418, -1565.6306) projected
  line L502 (3395.1418, -1565.6306) -> (3459.3022, -1565.6306) projected
  line L503 (3459.3022, -1565.6306) -> (3459.4292, -1565.6052) projected
  line L504 (3459.4292, -1565.6052) -> (3459.5816, -1565.6052) projected
  line L505 (3459.5816, -1565.6052) -> (3459.7086, -1565.5569) projected
  line L506 (3459.7086, -1565.5569) -> (3459.861, -1565.5341) projected
  line L507 (3459.861, -1565.5341) -> (3459.9626, -1565.463) projected
  line L508 (3459.9626, -1565.463) -> (3460.115, -1565.4147) projected
  line L509 (3460.115, -1565.4147) -> (3460.2166, -1565.3233) projected
  line L510 (3460.2166, -1565.3233) -> (3460.3436, -1565.2521) projected
  line L511 (3460.3436, -1565.2521) -> (3460.4198, -1565.1455) projected
  line L512 (3460.4198, -1565.1455) -> (3460.5214, -1565.054) projected
  line L513 (3460.5214, -1565.054) -> (3460.5976, -1564.9321) projected
  line L514 (3460.5976, -1564.9321) -> (3460.6992, -1564.8254) projected
  line L515 (3460.6992, -1564.8254) -> (3460.75, -1564.6908) projected
  line L516 (3460.75, -1564.6908) -> (3460.8262, -1564.5689) projected
  line L517 (3460.8262, -1564.5689) -> (3460.8262, -1564.4292) projected
  line L518 (3460.8262, -1564.4292) -> (3460.877, -1564.2971) projected
  line L519 (3460.877, -1564.2971) -> (3460.877, -1564.1574) projected
  line L520 (3460.877, -1564.1574) -> (3460.9024, -1564.0177) projected
  line L521 (3460.9024, -1564.0177) -> (3460.9024, -1563.0601) projected
  line L522 (3460.9024, -1563.0601) -> (3461.3342, -1560.9189) projected
  line L523 (3461.3342, -1560.9189) -> (3462.4518, -1559.2374) projected
  line L524 (3462.4518, -1559.2374) -> (3464.1282, -1558.1147) projected
  line L525 (3464.1282, -1558.1147) -> (3466.2872, -1557.688) projected
  line L526 (3466.2872, -1557.688) -> (3482.086, -1557.688) projected
  line L527 (3482.086, -1557.688) -> (3484.245, -1558.1147) projected
  line L528 (3484.245, -1558.1147) -> (3485.9214, -1559.2374) projected
  line L529 (3485.9214, -1559.2374) -> (3487.039, -1560.9189) projected
  line L530 (3487.039, -1560.9189) -> (3487.1406, -1561.4117) projected
  line L531 (3487.1406, -1561.4117) -> (3487.2168, -1561.6555) projected
  line L532 (3487.2168, -1561.6555) -> (3487.3184, -1561.9019) projected
  line L533 (3487.3184, -1561.9019) -> (3487.3184, -1561.9171) projected
  line L534 (3487.3184, -1561.9171) -> (3487.3438, -1561.9324) projected
  line L535 (3487.3438, -1561.9324) -> (3487.5216, -1562.1305) projected
  line L536 (3487.5216, -1562.1305) -> (3487.674, -1562.3311) projected
  line L537 (3487.674, -1562.3311) -> (3487.6994, -1562.3413) projected
  line L538 (3487.6994, -1562.3413) -> (3487.6994, -1562.354) projected
  line L539 (3487.6994, -1562.354) -> (3487.928, -1562.481) projected
  line L540 (3487.928, -1562.481) -> (3488.1566, -1562.6131) projected
  line L541 (3488.1566, -1562.6131) -> (3488.182, -1562.6156) projected
  line L542 (3488.182, -1562.6156) -> (3488.2074, -1562.6232) projected
  line L543 (3488.2074, -1562.6232) -> (3488.4614, -1562.6639) projected
  line L544 (3488.4614, -1562.6639) -> (3488.7154, -1562.7096) projected
  line L545 (3488.7154, -1562.7096) -> (3500.3486, -1562.7096) projected
  line L546 (3500.3486, -1562.7096) -> (3500.5772, -1562.669) projected
  line L547 (3500.5772, -1562.669) -> (3500.7804, -1562.6461) projected
  line L548 (3500.7804, -1562.6461) -> (3500.8312, -1562.6207) projected
  line L549 (3500.8312, -1562.6207) -> (3500.882, -1562.6131) projected
  line L550 (3500.882, -1562.6131) -> (3501.0852, -1562.4988) projected
  line L551 (3501.0852, -1562.4988) -> (3501.2884, -1562.3972) projected
  line L552 (3501.2884, -1562.3972) -> (3501.3392, -1562.3591) projected
  line L553 (3501.3392, -1562.3591) -> (3501.39, -1562.3311) projected
  line L554 (3501.39, -1562.3311) -> (3501.4408, -1562.2473) projected
  line L555 (3501.4408, -1562.2473) -> (3503.2442, -1561.0484) projected
  line L556 (3503.2442, -1561.0484) -> (3505.3778, -1560.6217) projected
  line L557 (3505.3778, -1560.6217) -> (3513.963, -1560.6217) projected
  line L558 (3513.963, -1560.6217) -> (3516.0966, -1561.0484) projected
  line L559 (3516.0966, -1561.0484) -> (3516.1982, -1561.117) projected
  line L560 (3516.1982, -1561.117) -> (3516.376, -1561.1958) projected
  line L561 (3516.376, -1561.1958) -> (3516.5538, -1561.2923) projected
  line L562 (3516.5538, -1561.2923) -> (3516.63, -1561.3075) projected
  line L563 (3516.63, -1561.3075) -> (3516.7062, -1561.3431) projected
  line L564 (3516.7062, -1561.3431) -> (3516.9094, -1561.3558) projected
  line L565 (3516.9094, -1561.3558) -> (3517.0872, -1561.3888) projected
  line L566 (3517.0872, -1561.3888) -> (3521.6084, -1561.3888) projected
  line L567 (3521.6084, -1561.3888) -> (3521.7862, -1561.3558) projected
  line L568 (3521.7862, -1561.3558) -> (3521.9894, -1561.3431) projected
  line L569 (3521.9894, -1561.3431) -> (3522.0656, -1561.3075) projected
  line L570 (3522.0656, -1561.3075) -> (3522.1418, -1561.2923) projected
  line L571 (3522.1418, -1561.2923) -> (3522.3196, -1561.1958) projected
  line L572 (3522.3196, -1561.1958) -> (3522.4974, -1561.117) projected
  line L573 (3522.4974, -1561.117) -> (3522.599, -1561.0484) projected
  line L574 (3522.599, -1561.0484) -> (3524.7326, -1560.6217) projected
  line L575 (3524.7326, -1560.6217) -> (3533.3178, -1560.6217) projected
  line L576 (3533.3178, -1560.6217) -> (3535.4514, -1561.0484) projected
  line L577 (3535.4514, -1561.0484) -> (3537.1278, -1562.1711) projected
  line L578 (3537.1278, -1562.1711) -> (3538.2454, -1563.8526) projected
  line L579 (3538.2454, -1563.8526) -> (3538.6772, -1565.9938) projected
  line L580 (3538.6772, -1565.9938) -> (3538.6772, -1573.2938) projected
  line L581 (3538.6772, -1573.2938) -> (3538.3724, -1574.9041) projected
  line L582 (3538.3724, -1574.9041) -> (3538.3724, -1574.9219) projected
  line L583 (3538.3724, -1574.9219) -> (3538.347, -1574.9397) projected
  line L584 (3538.347, -1574.9397) -> (3538.347, -1575.2013) projected
  line L585 (3538.347, -1575.2013) -> (3538.347, -1575.4655) projected
  line L586 (3538.347, -1575.4655) -> (3538.347, -1575.4807) projected
  line L587 (3538.347, -1575.4807) -> (3538.347, -1575.4985) projected
  line L588 (3538.347, -1575.4985) -> (3538.4642, -1575.7959) projected
  line L589 (3473.6532, -1464.3964) -> (3473.6532, -1467.358) projected
  line L590 (3473.6532, -1467.358) -> (3476.498, -1467.358) projected
  line L591 (3476.498, -1467.358) -> (3476.498, -1474.0001) projected
  line L592 (3476.498, -1474.0001) -> (3479.4698, -1474.0001) projected
  line L593 (3479.4698, -1474.0001) -> (3479.7238, -1473.7359) projected
  line L594 (3479.7238, -1473.7359) -> (3479.7238, -1466.7154) projected
  line L595 (3479.7238, -1466.7154) -> (3479.2412, -1465.5317) projected
  line L596 (3479.2412, -1465.5317) -> (3478.3268, -1464.6224) projected
  line L597 (3478.3268, -1464.6224) -> (3477.133, -1464.1322) projected
  line L598 (3477.133, -1464.1322) -> (3473.9326, -1464.1322) projected
  line L599 (3473.9326, -1464.1322) -> (3473.6532, -1464.3964) projected
  line L600 (3456.8892, -1464.6224) -> (3455.9748, -1465.5317) projected
  line L601 (3455.9748, -1465.5317) -> (3455.4922, -1466.7154) projected
  line L602 (3455.4922, -1466.7154) -> (3455.4922, -1473.7359) projected
  line L603 (3455.4922, -1473.7359) -> (3455.7462, -1474.0001) projected
  line L604 (3455.7462, -1474.0001) -> (3458.718, -1474.0001) projected
  line L605 (3458.718, -1474.0001) -> (3458.718, -1467.358) projected
  line L606 (3458.718, -1467.358) -> (3461.5374, -1467.358) projected
  line L607 (3461.5374, -1467.358) -> (3461.5374, -1464.3964) projected
  line L608 (3461.5374, -1464.3964) -> (3461.2834, -1464.1322) projected
  line L609 (3461.2834, -1464.1322) -> (3458.083, -1464.1322) projected
  line L610 (3458.083, -1464.1322) -> (3456.8892, -1464.6224) projected
  line L611 (3365.9826, -1575.7959) -> (3365.9826, -1567.5356) projected
  line L612 (3365.9826, -1567.5356) -> (3388.8426, -1567.5356) projected
  line L613 (3388.8426, -1567.5356) -> (3388.8426, -1570.7106) projected
  line L614 (3388.8426, -1570.7106) -> (3466.1348, -1570.7106) projected
  line L615 (3466.1348, -1570.7106) -> (3466.1348, -1562.9001) projected
  line L616 (3466.1348, -1562.9001) -> (3482.2384, -1562.9001) projected
  line L617 (3482.2384, -1562.9001) -> (3482.2384, -1567.7896) projected
  line L618 (3482.2384, -1567.7896) -> (3505.2254, -1567.7896) projected
  line L619 (3505.2254, -1567.7896) -> (3505.2254, -1565.8338) projected
  line L620 (3505.2254, -1565.8338) -> (3514.1154, -1565.8338) projected
  line L621 (3514.1154, -1565.8338) -> (3514.1154, -1566.4688) projected
  line L622 (3514.1154, -1566.4688) -> (3524.5802, -1566.4688) projected
  line L623 (3524.5802, -1566.4688) -> (3524.5802, -1565.8338) projected
  line L624 (3524.5802, -1565.8338) -> (3533.4702, -1565.8338) projected
  line L625 (3533.4702, -1565.8338) -> (3533.4702, -1573.4538) projected
  line L626 (3533.4702, -1573.4538) -> (3524.5802, -1573.4538) projected
  line L627 (3524.5802, -1573.4538) -> (3524.5802, -1572.8188) projected
  line L628 (3524.5802, -1572.8188) -> (3514.1154, -1572.8188) projected
  line L629 (3514.1154, -1572.8188) -> (3514.1154, -1573.4538) projected
  line L630 (3514.1154, -1573.4538) -> (3510.3054, -1573.4538) projected
  line L631 (3510.3054, -1573.4538) -> (3510.026, -1573.6138) projected
  line L632 (3510.026, -1573.6138) -> (3509.6958, -1573.8526) projected
  line L633 (3509.6958, -1573.8526) -> (3509.5688, -1573.8881) projected
  line L634 (3509.5688, -1573.8881) -> (3509.4418, -1573.9593) projected
  line L635 (3509.4418, -1573.9593) -> (3509.0354, -1574.0329) projected
  line L636 (3509.0354, -1574.0329) -> (3508.629, -1574.1396) projected
  line L637 (3508.629, -1574.1396) -> (3508.4766, -1574.1269) projected
  line L638 (3508.4766, -1574.1269) -> (3508.4258, -1574.1396) projected
  line L639 (3508.4258, -1574.1396) -> (3482.2384, -1574.1396) projected
  line L640 (3482.2384, -1574.1396) -> (3482.2384, -1575.7959) projected
  line L641 (3232.2262, -1452.1739) -> (3232.2262, -1452.0316) projected
  line L642 (3232.2262, -1452.0316) -> (3233.801, -1443.0832) projected
  line L643 (3233.801, -1443.0832) -> (3234.0042, -1442.5574) projected
  line L644 (3234.0042, -1442.5574) -> (3238.1952, -1435.3057) projected
  line L645 (3238.1952, -1435.3057) -> (3238.3984, -1435.0721) projected
  line L646 (3238.3984, -1435.0721) -> (3238.5508, -1434.8765) projected
  line L647 (3238.5508, -1434.8765) -> (3244.977, -1429.4942) projected
  line L648 (3244.977, -1429.4942) -> (3245.4596, -1429.2148) projected
  line L649 (3245.4596, -1429.2148) -> (3253.6638, -1426.2278) projected
  line L650 (3253.6638, -1426.2278) -> (3253.867, -1426.1922) projected
  line L651 (3253.867, -1426.1922) -> (3254.0702, -1426.1363) projected
  line L652 (3254.0702, -1426.1363) -> (3258.2612, -1425.768) projected
  line L653 (3258.2612, -1425.768) -> (3258.3374, -1425.7757) projected
  line L654 (3258.3374, -1425.7757) -> (3258.4136, -1425.763) projected
  line L655 (3258.4136, -1425.763) -> (3837.9908, -1425.763) projected
  line L656 (3837.9908, -1425.763) -> (3838.1432, -1425.7884) projected
  line L657 (3838.1432, -1425.7884) -> (3838.2702, -1425.7884) projected
  line L658 (3838.2702, -1425.7884) -> (3847.2364, -1427.3657) projected
  line L659 (3847.2364, -1427.3657) -> (3847.7444, -1427.5562) projected
  line L660 (3847.7444, -1427.5562) -> (3855.0088, -1431.7447) projected
  line L661 (3855.0088, -1431.7447) -> (3855.2374, -1431.9402) projected
  line L662 (3855.2374, -1431.9402) -> (3855.4406, -1432.1028) projected
  line L663 (3855.4406, -1432.1028) -> (3860.8254, -1438.5188) projected
  line L664 (3860.8254, -1438.5188) -> (3861.1048, -1439.004) projected
  line L665 (3861.1048, -1439.004) -> (3864.0766, -1447.2082) projected
  line L666 (3864.0766, -1447.2082) -> (3864.1274, -1447.4165) projected
  line L667 (3864.1274, -1447.4165) -> (3864.1782, -1447.6197) projected
  line L668 (3864.1782, -1447.6197) -> (3864.5338, -1451.8208) projected
  line L669 (3864.5338, -1451.8208) -> (3864.5592, -1575.7959) projected
  line L670 (3864.5592, -1575.7959) -> (3232.2008, -1575.7959) projected
  line L671 (3232.2008, -1575.7959) -> (3232.2008, -1452.311) projected
  line L672 (3232.2008, -1452.311) -> (3232.2262, -1452.1739) projected
  circle A0 centre (3312.8966, -1487.0938) radius 4.8387 projected
  circle A1 centre (3312.8966, -1487.0938) radius 4.8387 projected
  circle A2 centre (3248.3806, -1483.868) radius 4.8387 projected
  circle A3 centre (3248.3806, -1483.868) radius 4.8387 projected
  circle A4 centre (3248.3806, -1464.5132) radius 4.8387 projected
  circle A5 centre (3248.3806, -1464.5132) radius 4.8387 projected
  circle A6 centre (3248.3806, -1445.1584) radius 4.8387 projected
  circle A7 centre (3248.3806, -1445.1584) radius 4.8387 projected
  circle A8 centre (3267.7354, -1445.1584) radius 4.8387 projected
  circle A9 centre (3267.7354, -1445.1584) radius 4.8387 projected
  circle A10 centre (3287.0902, -1445.1584) radius 4.8387 projected
  circle A11 centre (3287.0902, -1445.1584) radius 4.8387 projected
  circle A12 centre (3312.8966, -1464.5132) radius 4.8387 projected
  circle A13 centre (3248.3806, -1503.2228) radius 4.8387 projected
  circle A14 centre (3312.8966, -1506.4486) radius 4.8387 projected
  circle A15 centre (3312.8966, -1506.4486) radius 4.8387 projected
  circle A16 centre (3312.8966, -1525.8034) radius 4.8387 projected
  circle A17 centre (3312.8966, -1525.8034) radius 4.8387 projected
  circle A18 centre (3312.8966, -1545.1582) radius 4.8387 projected
  circle A19 centre (3312.8966, -1545.1582) radius 4.8387 projected
  circle A20 centre (3312.8966, -1564.513) radius 4.8387 projected
  circle A21 centre (3312.8966, -1564.513) radius 4.8387 projected
  circle A22 centre (3248.3806, -1522.5776) radius 4.8387 projected
  circle A23 centre (3248.3806, -1522.5776) radius 4.8387 projected
  circle A24 centre (3248.3806, -1541.9324) radius 4.8387 projected
  circle A25 centre (3248.3806, -1541.9324) radius 4.8387 projected
  circle A26 centre (3248.3806, -1561.2872) radius 4.8387 projected
  circle A27 centre (3248.3806, -1561.2872) radius 4.8387 projected
  circle A28 centre (3248.3806, -1503.2228) radius 4.8387 projected
  circle A29 centre (3383.8642, -1445.1584) radius 4.8387 projected
  circle A30 centre (3383.8642, -1445.1584) radius 4.8387 projected
  circle A31 centre (3364.5094, -1445.1584) radius 4.8387 projected
  circle A32 centre (3364.5094, -1445.1584) radius 4.8387 projected
  circle A33 centre (3345.1546, -1445.1584) radius 4.8387 projected
  circle A34 centre (3345.1546, -1445.1584) radius 4.8387 projected
  circle A35 centre (3325.7998, -1445.1584) radius 4.8387 projected
  circle A36 centre (3325.7998, -1445.1584) radius 4.8387 projected
  circle A37 centre (3312.8966, -1464.5132) radius 4.8387 projected
  circle A38 centre (3467.735, -1545.1582) radius 4.8387 projected
  circle A39 centre (3467.735, -1545.1582) radius 4.8387 projected
  circle A40 centre (3412.8964, -1545.1582) radius 4.8387 projected
  circle A41 centre (3412.8964, -1545.1582) radius 4.8387 projected
  circle A42 centre (3438.7028, -1545.1582) radius 4.8387 projected
  circle A43 centre (3438.7028, -1545.1582) radius 4.8387 projected
  circle A44 centre (3403.219, -1445.1584) radius 4.8387 projected
  circle A45 centre (3403.219, -1445.1584) radius 4.8387 projected
  circle A46 centre (3422.5738, -1445.1584) radius 4.8387 projected
  circle A47 centre (3422.5738, -1445.1584) radius 4.8387 projected
  circle A48 centre (3441.9286, -1445.1584) radius 4.8387 projected
  circle A49 centre (3441.9286, -1445.1584) radius 4.8387 projected
  circle A50 centre (3306.445, -1445.1584) radius 4.8387 projected
  circle A51 centre (3306.445, -1445.1584) radius 4.8387 projected
  line L673 (3538.4486, -1575.7449) -> (3538.347, -1575.4985) projected
  line L674 (3698.3924, -1575.7959) -> (3698.3924, -1574.1396) projected
  line L675 (3698.3924, -1574.1396) -> (3721.3286, -1574.1396) projected
  line L676 (3721.3286, -1574.1396) -> (3721.9128, -1574.0355) projected
  line L677 (3721.9128, -1574.0355) -> (3722.497, -1574.1396) projected
  line L678 (3722.497, -1574.1396) -> (3737.483, -1574.1396) projected
  line L679 (3737.483, -1574.1396) -> (3737.483, -1574.7746) projected
  line L680 (3737.483, -1574.7746) -> (3746.373, -1574.7746) projected
  line L681 (3746.373, -1574.7746) -> (3746.373, -1574.1396) projected
  line L682 (3746.373, -1574.1396) -> (3756.8378, -1574.1396) projected
  line L683 (3756.8378, -1574.1396) -> (3756.8378, -1574.7746) projected
  line L684 (3756.8378, -1574.7746) -> (3765.7278, -1574.7746) projected
  line L685 (3765.7278, -1574.7746) -> (3765.7278, -1567.1546) projected
  line L686 (3765.7278, -1567.1546) -> (3756.8378, -1567.1546) projected
  line L687 (3756.8378, -1567.1546) -> (3756.8378, -1567.7896) projected
  line L688 (3756.8378, -1567.7896) -> (3746.373, -1567.7896) projected
  line L689 (3746.373, -1567.7896) -> (3746.373, -1567.1546) projected
  line L690 (3746.373, -1567.1546) -> (3737.483, -1567.1546) projected
  line L691 (3737.483, -1567.1546) -> (3737.483, -1567.7896) projected
  line L692 (3737.483, -1567.7896) -> (3722.497, -1567.7896) projected
  line L693 (3722.497, -1567.7896) -> (3721.9128, -1567.8937) projected
  line L694 (3721.9128, -1567.8937) -> (3721.3286, -1567.7896) projected
  line L695 (3721.3286, -1567.7896) -> (3698.3924, -1567.7896) projected
  line L696 (3698.3924, -1567.7896) -> (3698.3924, -1562.9001) projected
  line L697 (3698.3924, -1562.9001) -> (3693.4902, -1562.9001) projected
  line L698 (3693.4902, -1562.9001) -> (3693.4902, -1556.4815) projected
  line L699 (3693.4902, -1556.4815) -> (3693.4902, -1556.4129) projected
  line L700 (3693.4902, -1556.4129) -> (3693.4902, -1556.2732) projected
  line L701 (3693.4902, -1556.2732) -> (3693.3886, -1555.8694) projected
  line L702 (3693.3886, -1555.8694) -> (3693.3124, -1555.4604) projected
  line L703 (3693.3124, -1555.4604) -> (3693.2362, -1555.3385) projected
  line L704 (3693.2362, -1555.3385) -> (3693.2108, -1555.2039) projected
  line L705 (3693.2108, -1555.2039) -> (3692.9568, -1554.861) projected
  line L706 (3692.9568, -1554.861) -> (3692.7536, -1554.5003) projected
  line L707 (3692.7536, -1554.5003) -> (3692.652, -1554.4114) projected
  line L708 (3692.652, -1554.4114) -> (3692.6012, -1554.353) projected
  line L709 (3692.6012, -1554.353) -> (3655.314, -1517.0582) projected
  line L710 (3655.314, -1517.0582) -> (3655.2632, -1517.0175) projected
  line L711 (3655.2632, -1517.0175) -> (3655.1616, -1516.9109) projected
  line L712 (3655.1616, -1516.9109) -> (3654.806, -1516.7026) projected
  line L713 (3654.806, -1516.7026) -> (3654.4758, -1516.4638) projected
  line L714 (3654.4758, -1516.4638) -> (3654.3234, -1516.4283) projected
  line L715 (3654.3234, -1516.4283) -> (3654.1964, -1516.3571) projected
  line L716 (3654.1964, -1516.3571) -> (3653.79, -1516.2835) projected
  line L717 (3653.79, -1516.2835) -> (3653.3836, -1516.1768) projected
  line L718 (3653.3836, -1516.1768) -> (3653.2566, -1516.1895) projected
  line L719 (3653.2566, -1516.1895) -> (3653.1804, -1516.1768) projected
  line L720 (3653.1804, -1516.1768) -> (3537.9914, -1516.1768) projected
  line L721 (3537.9914, -1516.1768) -> (3537.9914, -1507.9218) projected
  line L722 (3537.9914, -1507.9218) -> (3525.2914, -1507.9218) projected
  line L723 (3525.2914, -1507.9218) -> (3525.2914, -1530.7818) projected
  line L724 (3525.2914, -1530.7818) -> (3537.9914, -1530.7818) projected
  line L725 (3537.9914, -1530.7818) -> (3537.9914, -1522.5268) projected
  line L726 (3537.9914, -1522.5268) -> (3651.8088, -1522.5268) projected
  line L727 (3651.8088, -1522.5268) -> (3687.1402, -1557.8658) projected
  line L728 (3687.1402, -1557.8658) -> (3687.1402, -1562.9001) projected
  line L729 (3687.1402, -1562.9001) -> (3682.238, -1562.9001) projected
  line L730 (3682.238, -1562.9001) -> (3682.238, -1575.7959) projected
  circle A52 centre (3577.4122, -1548.384) radius 4.8387 projected
  circle A53 centre (3577.4122, -1548.384) radius 4.8387 projected
  circle A54 centre (3548.38, -1548.384) radius 4.8387 projected
  circle A55 centre (3548.38, -1548.384) radius 4.8387 projected
  circle A56 centre (3635.4766, -1548.384) radius 4.8387 projected
  circle A57 centre (3635.4766, -1548.384) radius 4.8387 projected
  circle A58 centre (3606.4444, -1548.384) radius 4.8387 projected
  circle A59 centre (3606.4444, -1548.384) radius 4.8387 projected
  line L731 (3864.5338, -1451.8208) -> (3864.5338, -1451.8894) projected
  line L732 (3864.5338, -1451.8894) -> (3864.5592, -1451.9605) projected
  circle A60 centre (3596.767, -1445.1584) radius 4.8387 projected
  circle A61 centre (3596.767, -1445.1584) radius 4.8387 projected
  circle A62 centre (3616.1218, -1445.1584) radius 4.8387 projected
  circle A63 centre (3616.1218, -1445.1584) radius 4.8387 projected